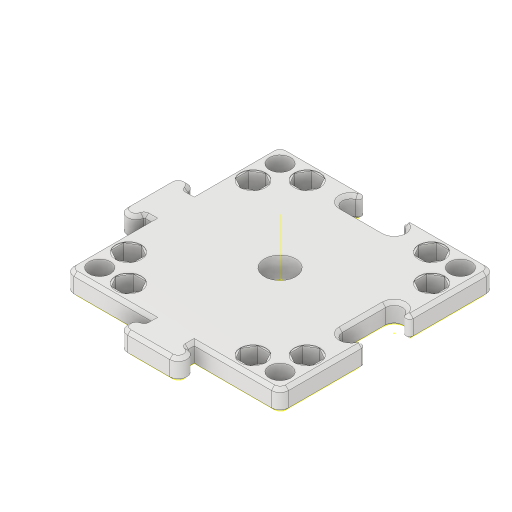
# Autodesk Inventor part: 10_Base_puzzle_syringetip_7.3mm
Saved by Autodesk Inventor 2024.1 (Build 281209000, 209)
## iProperties
Created: 2017-06-20
Part Number: 10_Base_puzzle_syringetip_7.3mm
Material: Generisch
Document SubType Name: Modeling
Designer: diederichbenedict
Density: 1 g/cm^3
Appearance: Weiß
Mass: 5.4697 g
Surface Area: 48.9743 cm^2
Volume: 5.4697 cm^3
Catalog Web Link: isInjectionmolded
Vendor: openUC2
d_part: 50,000 mm
d_o: 40,000 mm
d_i: 40,000 mm
Author: diederichbenedict
Autodesk Inventor part; units mm, degrees
ref_plane "YZ Plane" through (0, 0, 0) normal (1, 0, 0) x (0, 1, 0)
ref_plane "XZ Plane" through (0, 0, 0) normal (0, 1, 0) x (-1, 0, 0)
ref_plane "XY Plane" through (0, 0, 0) normal (0, 0, 1) x (1, 0, 0)
sketch "Skizze1" plane through (0, 0, 0) normal (0, 0, 1) x (1, 0, 0)
  line L0 (-17, 0) -> (-25, 0)
  line L1 (-25, 0) -> (-25, -23)
  line L2 (-23, -25) -> (0, -25)
  line L3 (0, -25) -> (0, -17)
  line L4 (-17, 0) -> (-17, -15)
  line L5 (-15, -17) -> (0, -17)
  arc A0 (-25, -23) -> (-23, -25) centre (-23, -23) ccw
  circle A1 centre (-20.8, -14.5) radius 2.55 construction
  circle A2 centre (-14.5, -20.8) radius 2.55 construction
  arc A3 (-17, -15) -> (-15, -17) centre (-15, -15) ccw
  circle A4 centre (-14.5, -20.8) radius 2.55 construction
  circle A5 centre (-20.8, -14.5) radius 2.55 construction
  line L6 (-30.4971, 0) -> (5.0828, 0) construction
  line L7 (0, -30.4971) -> (0, 5.0828) construction
  line L8 (-18.25, -13.0278) -> (-18.25, -15.9722)
  line L9 (-18.25, -15.9722) -> (-20.8, -17.4445)
  line L10 (-20.8, -17.4445) -> (-23.35, -15.9722)
  line L11 (-23.35, -15.9722) -> (-23.35, -13.0278)
  line L12 (-23.35, -13.0278) -> (-20.8, -11.5555)
  line L13 (-20.8, -11.5555) -> (-18.25, -13.0278)
  line L14 (-15.9722, -18.25) -> (-13.0278, -18.25)
  line L15 (-13.0278, -18.25) -> (-11.5555, -20.8)
  line L16 (-11.5555, -20.8) -> (-13.0278, -23.35)
  line L17 (-13.0278, -23.35) -> (-15.9722, -23.35)
  line L18 (-15.9722, -23.35) -> (-17.4445, -20.8)
  line L19 (-17.4445, -20.8) -> (-15.9722, -18.25)
  point P0 (-25, -25)
  point P1 (-17, -17)
  dimension "d278" = 25
  dimension "d279" = 25
  dimension "d2" = 8
  dimension "d281" = 8
  dimension "d282" = 2
  dimension "d286" = 5.1
  dimension "d_hole" = 5.1
  dimension "d290" = 20.8
  dimension "d" = 20.8
  dimension "d292" = 2
  dimension "d313" = 6.3
  dimension "d314" = 6.3
  dimension "d331" = 0
  dimension "d332" = 0
  constraints: 36 end point, 6 centre point, 6 tangent, 5 coincident, 4 parallel, 4 point on circle, 4 point on line, 2 collinear, 1 horizontal, 1 perpendicular, 26 other
  measures "d278" distance of L2.end point (-25, -25)
  measures "d279" distance of point (-25, -25) L0.end
  measures "d2" distance between parallel lines of L4 L1
  measures "d281" distance between parallel lines of L2 L5
  measures "d282" radius of A0
  measures "d286" diameter of A1
  measures "d_hole" diameter of A2
  measures "d290" distance from line of L0 A2.centre
  measures "d" distance from line of L3 A1.centre
  measures "d292" radius of A3
  measures "d313" horizontal distance of A1.centre A2.centre
  measures "d314" horizontal distance of A1.centre A2.centre
  measures "d331" radial gap between concentric circles of A2 A4
  measures "d332" radial gap between concentric circles of A1 A5
extrude "Extrusion1" add sketch "Skizze1" along normal blind 5
mirror "Mirror6" about plane through (-17, 0, 0) normal (0, 1, 0) of "Extrusion1"
mirror "Mirror7" about plane through (0, -25, 0) normal (1, 0, 0) of "Extrusion1", "Mirror6"
sketch "Sketch26" plane through (0, 0, 5) normal (0, 0, 1) x (1, 0, 0)
  line L0 (23, 25) -> (-23, 25) projected
  arc A0 (-23, 25) -> (-25, 23) centre (-23, 23) ccw projected
  line L1 (-25, -23) -> (-25, 23) projected
  arc A1 (-25, -23) -> (-23, -25) centre (-23, -23) ccw projected
  line L2 (-23, -25) -> (23, -25) projected
  arc A2 (23, -25) -> (25, -23) centre (23, -23) ccw projected
  line L3 (25, 23) -> (25, -23) projected
  arc A3 (25, 23) -> (23, 25) centre (23, 23) ccw projected
  line L4 (15, 17) -> (-15, 17) projected
  arc A4 (17, 15) -> (15, 17) centre (15, 15) ccw projected
  line L5 (17, 15) -> (17, -15) projected
  arc A5 (15, -17) -> (17, -15) centre (15, -15) ccw projected
  line L6 (-15, -17) -> (15, -17) projected
  arc A6 (-17, -15) -> (-15, -17) centre (-15, -15) ccw projected
  line L7 (-17, -15) -> (-17, 15) projected
  arc A7 (-15, 17) -> (-17, 15) centre (-15, 15) ccw projected
  line L8 (-25, -23) -> (-25, 23) projected
  line L9 (-28.6, -6.9) -> (-28.6, -6.9)
  line L10 (-30.6, -4.9) -> (-30.6, 4.9)
  line L11 (-28.6, 6.9) -> (-28.6, 6.9)
  line L12 (-25, 16.8311) -> (-25, -7)
  line L13 (-26.3774, 5) -> (-25, 5)
  line L14 (-25, -5) -> (-26.3774, -5)
  arc A8 (-30.6, -4.9) -> (-28.6, -6.9) centre (-28.6, -4.9) ccw
  arc A9 (-28.6, -6.9) -> (-26.6243, -5.2111) centre (-28.6, -4.9) ccw
  arc A10 (-28.6, 6.9) -> (-30.6, 4.9) centre (-28.6, 4.9) ccw
  arc A11 (-26.6243, 5.2111) -> (-28.6, 6.9) centre (-28.6, 4.9) ccw
  arc A12 (-26.3774, -5) -> (-26.6243, -5.2111) centre (-26.3774, -5.25) ccw
  arc A13 (-26.6243, 5.2111) -> (-26.3774, 5) centre (-26.3774, 5.25) ccw
  line L15 (-42.4199, 0) -> (36.7199, 0) projected
  point P0 (0, 0)
  point P1 (-24.0313, 1.861)
  point P2 (-25, -5)
  point P3 (-25, 5)
  point P4 (-28.6, 6.9)
  dimension "d293" = 5.6
  dimension "d300" = 2
  dimension "d301" = 0.25
  dimension "d365" = 6.9
  dimension "d367" = 6.9
  dimension "d385" = 5
  dimension "d386" = 5
  constraints: 12 end point, 12 point on circle, 10 tangent, 6 centre point, 4 equal radius, 3 parallel, 2 coincident, 2 point on line, 1 horizontal, 1 perpendicular, 1 other
  measures "d293" distance between parallel lines of L1 L10
  measures "d300" radius of A8
  measures "d301" radius of A12
  measures "d385" distance of the line from the sketch origin of L14
  measures "d386" distance of the line from the sketch origin of L13
extrude "Extrusion13" add sketch "Sketch26" against normal up to surface (5 mm away) contours L1 L15 L10 A10 A11 A13 L13 | L1 L14 A12 A9 A8 L10 L15
sketch "Sketch28" plane through (0, 0, 5) normal (0, 0, 1) x (1, 0, 0)
  line L0 (-42.0864, 0) -> (37.3113, 0) construction
  line L1 (23, 25) -> (-23, 25) projected
  arc A0 (-23, 25) -> (-25, 23) centre (-23, 23) ccw projected
  line L2 (-25, 5) -> (-25, 23) projected
  arc A1 (-25, -23) -> (-23, -25) centre (-23, -23) ccw projected
  line L3 (-23, -25) -> (23, -25) projected
  arc A2 (23, -25) -> (25, -23) centre (23, -23) ccw projected
  line L4 (25, 23) -> (25, -23) projected
  arc A3 (25, 23) -> (23, 25) centre (23, 23) ccw projected
  line L5 (15, 17) -> (-15, 17) projected
  arc A4 (17, 15) -> (15, 17) centre (15, 15) ccw projected
  line L6 (17, 15) -> (17, -15) projected
  arc A5 (15, -17) -> (17, -15) centre (15, -15) ccw projected
  line L7 (-15, -17) -> (15, -17) projected
  arc A6 (-17, -15) -> (-15, -17) centre (-15, -15) ccw projected
  line L8 (-17, -15) -> (-17, 15) projected
  arc A7 (-15, 17) -> (-17, 15) centre (-15, 15) ccw projected
  line L9 (24.4624, 5.1058) -> (23.9221, 5.1058) construction
  line L10 (19.1833, 5.0625) -> (23.3833, 5.0625) construction
  line L11 (19.1833, 5.0625) -> (23.3833, 5.0625) construction
  line L12 (23.3833, 5.0625) -> (23.4138, 5.032) construction
  line L13 (23.3833, 5.0625) -> (23.7431, 5.0625) construction
  line L14 (25, 5) -> (25, 0.1058)
  line L15 (25, 23) -> (25, -23) projected
  line L16 (24.4624, 5.1058) -> (25, 5.6434) construction
  line L17 (25, 5) -> (25.2369, 5) construction
  line L18 (25, 5.6434) -> (25, 5)
  line L19 (-25, 5) -> (-26.3774, 5) construction
  arc A8 (-26.6243, 5.2111) -> (-26.3774, 5) centre (-26.3774, 5.25) ccw construction
  arc A9 (-26.6243, 5.2111) -> (-30.6, 4.9) centre (-28.6, 4.9) ccw construction
  line L20 (-30.6, 4.9) -> (-30.6, -4.9) construction
  arc A10 (-30.6, -4.9) -> (-26.6243, -5.2111) centre (-28.6, -4.9) ccw construction
  arc A11 (-26.3774, -5) -> (-26.6243, -5.2111) centre (-26.3774, -5.25) ccw construction
  line L21 (-26.3774, -5) -> (-25, -5) construction
  line L22 (-25, -23) -> (-25, -5) projected
  line L23 (24.4624, -5.1058) -> (23.9221, -5.1058) construction
  line L24 (19.1833, -5.0625) -> (23.3833, -5.0625) construction
  line L25 (19.1833, -5.0625) -> (23.3833, -5.0625) construction
  line L26 (23.3833, -5.0625) -> (23.4138, -5.032) construction
  line L27 (23.3833, -5.0625) -> (23.7431, -5.0625) construction
  line L28 (25, -5) -> (25, 0.1058)
  line L29 (24.4624, -5.1058) -> (25, -5.6434) construction
  line L30 (25, -5) -> (25.2369, -5) construction
  line L31 (25, -5.6434) -> (25, -5)
  line L32 (21.3, -6.95) -> (21.3, -6.95) construction
  line L33 (19.3, -4.95) -> (19.3, 5.05) construction
  line L34 (21.3, 7.05) -> (21.3, 7.05) construction
  line L35 (23.5226, 5.1498) -> (25, 5.1497) construction
  line L36 (25, -5.0501) -> (23.5226, -5.05) construction
  arc A12 (19.3, -4.95) -> (21.3, -6.95) centre (21.3, -4.95) ccw construction
  arc A13 (21.3, -6.95) -> (23.2757, -5.2611) centre (21.3, -4.95) ccw construction
  arc A14 (21.3, 7.05) -> (19.3, 5.05) centre (21.3, 5.05) ccw construction
  arc A15 (23.2757, 5.3609) -> (21.3, 7.05) centre (21.3, 5.05) ccw construction
  arc A16 (23.5226, -5.05) -> (23.2757, -5.2611) centre (23.5226, -5.3) ccw construction
  arc A17 (23.2757, 5.3609) -> (23.5226, 5.1498) centre (23.5226, 5.3998) ccw construction
  line L37 (-30.6, 4.9) -> (-30.6, -4.9) projected
  line L38 (-25, 5) -> (-26.3774, 5) projected
  line L39 (-25, 5) -> (-26.3774, 5)
  arc A18 (-26.6243, 5.2111) -> (-26.3774, 5) centre (-26.3774, 5.25) ccw projected
  arc A19 (-26.6243, 5.2111) -> (-26.3774, 5) centre (-26.3774, 5.25) ccw
  arc A20 (-26.6243, 5.2111) -> (-30.6, 4.9) centre (-28.6, 4.9) ccw
  line L40 (-30.6, 4.9) -> (-30.6, 0)
  line L41 (25, 5.1497) -> (23.4675, 5.1498)
  arc A21 (23.4675, 5.1498) -> (19.55, 5.05) centre (21.51, 5.05) ccw
  line L42 (19.55, 5.05) -> (19.55, 0)
  line L43 (24.4624, -5.1058) -> (23.9221, -5.1058) construction
  line L44 (19.1833, -5.0625) -> (23.3833, -5.0625) construction
  line L45 (19.1833, -5.0625) -> (23.3833, -5.0625) construction
  line L46 (23.3833, -5.0625) -> (23.4138, -5.032) construction
  line L47 (23.3833, -5.0625) -> (23.7431, -5.0625) construction
  line L48 (25, -5) -> (25, -0.1058)
  line L49 (24.4624, -5.1058) -> (25, -5.6434) construction
  line L50 (25, -5) -> (25.2369, -5) construction
  line L51 (25, -5.6434) -> (25, -5)
  arc A22 (23.5226, -5.1498) -> (23.2757, -5.3609) centre (23.5226, -5.3998) ccw construction
  arc A23 (21.3, -7.05) -> (23.2757, -5.3609) centre (21.3, -5.05) ccw construction
  line L52 (23.5226, -5.1498) -> (25, -5.1497) construction
  arc A24 (19.3, -5.05) -> (21.3, -7.05) centre (21.3, -5.05) ccw construction
  line L53 (25, -5.1497) -> (23.4675, -5.1498)
  arc A25 (19.55, -5.05) -> (23.4675, -5.1498) centre (21.51, -5.05) ccw
  arc A26 (23.4675, -5.1498) -> (23.4675, -5.1498) centre (23.3175, -5.15) ccw
  line L54 (19.55, -5.05) -> (19.55, 0)
  line L55 (19.55, 0) -> (25, 0)
  point P0 (23.3495, 5.1058)
  point P1 (23.3495, -5.1058)
  point P2 (25, -7)
  point P3 (25.9687, 1.861)
  point P4 (23.3495, -5.1058)
  point P5 (25.9687, -1.861)
  point P6 (23.4675, -5.1498)
  dimension "d14" = 0
  dimension "d20" = 0
  dimension "d369" = 4.2
  dimension "d370" = 0
  dimension "d380" = 45
  dimension "d387" = 2
  dimension "d388" = 0.25
  dimension "d391" = 0.1
  dimension "d392" = 5.05
  dimension "d393" = 5.05
  dimension "d394" = 1.96
  dimension "d396" = 5.45
  dimension "d397" = 7.05
  constraints: 80 end point, 30 symmetric about line, 28 point on circle, 14 centre point, 14 tangent, 8 point on line, 5 horizontal, 4 collinear, 4 equal radius, 3 coincident, 2 parallel, 2 perpendicular, 1 midpoint, 4 other
  measures "d369" distance of L10.start L10.end
  measures "d370" distance between parallel lines of L10 L11
  measures "d380" angle of L17 L16
  measures "d387" radius of A12
  measures "d388" radius of A16
  measures "d391" distance from line of L35 A15.centre
  measures "d392" distance from line of L0 A15.centre
  measures "d393" distance from line of L0 A21.centre
  measures "d394" radius of A21
  measures "d396" distance between parallel lines of L4 L42
  measures "d397" distance from line of L0 L34.end
extrude "Extrusion14" cut sketch "Sketch28" against normal blind 10 contours L4 L55 L42 A21 L41 | A26 | L4 L53 A25 L54 L55
pattern_circular "Circular Pattern6" count 2 over 90 about axis through (0, 0, 5) along (0, 0, 1) of "Extrusion14", "Extrusion13"
sketch "Sketch29" plane through (0, 0, 5) normal (0, 0, 1) x (1, 0, 0)
  arc A0 (-23, 25) -> (-25, 23) centre (-23, 23) ccw projected
  line L0 (-25, 5) -> (-25, 23) projected
  arc A1 (-25, -23) -> (-23, -25) centre (-23, -23) ccw projected
  line L1 (-23, -25) -> (-5, -25) projected
  arc A2 (23, -25) -> (25, -23) centre (23, -23) ccw projected
  arc A3 (25, 23) -> (23, 25) centre (23, 23) ccw projected
  line L2 (15, 17) -> (-15, 17) projected
  arc A4 (17, 15) -> (15, 17) centre (15, 15) ccw projected
  line L3 (17, 15) -> (17, -15) projected
  arc A5 (15, -17) -> (17, -15) centre (15, -15) ccw projected
  line L4 (-15, -17) -> (15, -17) projected
  arc A6 (-17, -15) -> (-15, -17) centre (-15, -15) ccw projected
  line L5 (-17, -15) -> (-17, 15) projected
  arc A7 (-15, 17) -> (-17, 15) centre (-15, 15) ccw projected
  circle A8 centre (-22, 0) radius 3.89
  circle A9 centre (0, -22) radius 2.9259
  line L6 (-41.9755, 0) -> (36.6458, 0) construction
  line L7 (0, -41.9755) -> (0, 36.6458) construction
  line L8 (25, -5.1497) -> (25, -23) projected
  line L9 (-5.1497, 25) -> (-23, 25) projected
  line L10 (-25, 5) -> (-26.3774, 5) projected
  arc A10 (-26.6243, 5.2111) -> (-26.3774, 5) centre (-26.3774, 5.25) ccw projected
  arc A11 (-26.6243, 5.2111) -> (-30.6, 4.9) centre (-28.6, 4.9) ccw projected
  line L11 (-30.6, 4.9) -> (-30.6, -4.9) projected
  arc A12 (-30.6, -4.9) -> (-26.6243, -5.2111) centre (-28.6, -4.9) ccw projected
  arc A13 (-26.3774, -5) -> (-26.6243, -5.2111) centre (-26.3774, -5.25) ccw projected
  line L12 (-26.3774, -5) -> (-25, -5) projected
  line L13 (-25, -23) -> (-25, -5) projected
  line L14 (-5, -25) -> (-5, -26.3774) projected
  arc A14 (-5.2111, -26.6243) -> (-5, -26.3774) centre (-5.25, -26.3774) ccw projected
  arc A15 (-5.2111, -26.6243) -> (-4.9, -30.6) centre (-4.9, -28.6) ccw projected
  line L15 (-4.9, -30.6) -> (4.9, -30.6) projected
  arc A16 (4.9, -30.6) -> (5.2111, -26.6243) centre (4.9, -28.6) ccw projected
  arc A17 (5, -26.3774) -> (5.2111, -26.6243) centre (5.25, -26.3774) ccw projected
  line L16 (5, -26.3774) -> (5, -25) projected
  line L17 (5, -25) -> (23, -25) projected
  line L18 (-5.1498, 23.4675) -> (-5.1497, 25) projected
  line L19 (25, -5.1497) -> (23.4675, -5.1498) projected
  arc A18 (19.55, -5.05) -> (23.4675, -5.1498) centre (21.51, -5.05) ccw projected
  line L20 (19.55, -5.05) -> (19.55, 5.05) projected
  arc A19 (23.4675, 5.1498) -> (19.55, 5.05) centre (21.51, 5.05) ccw projected
  line L21 (23.4675, 5.1498) -> (25, 5.1497) projected
  line L22 (25, 23) -> (25, 5.1497) projected
  line L23 (23, 25) -> (5.1497, 25) projected
  line L24 (5.1497, 25) -> (5.1498, 23.4675) projected
  arc A20 (5.05, 19.55) -> (5.1498, 23.4675) centre (5.05, 21.51) ccw projected
  line L25 (5.05, 19.55) -> (-5.05, 19.55) projected
  arc A21 (-5.1498, 23.4675) -> (-5.05, 19.55) centre (-5.05, 21.51) ccw projected
  point P0 (0, 0)
  dimension "d319" = 7.78
  dimension "d320" = 5
  dimension "d322" = 5
  constraints: 2 centre point, 2 point on line, 1 coincident
  measures "d319" diameter of A8
  measures "d320" distance from line of A8.centre L5
  measures "d322" distance from line of L4 A9.centre
hole "Hole7" [suppressed]
chamfer "Fase4" [suppressed]
fillet "Rundung5" radius 0.85 8 edges at (25, 5.1497, 2.5) (5.1497, 25, 2.5) (-5.1498, 23.4675, 2.5) (5.1498, 23.4675, 2.5) (23.4675, 5.1498, 2.5) (23.4675, -5.1498, 2.5) (25, -5.1497, 2.5) (-5.1497, 25, 2.5)
sketch "Skizze36" plane through (0, 0, 5) normal (0, 0, 1) x (1, 0, 0)
  line L0 (25, -6.0125) -> (25, -23) projected
  arc A0 (25, 23) -> (23, 25) centre (23, 23) ccw projected
  line L1 (23, 25) -> (6.0125, 25) projected
  line L2 (-6.0125, 25) -> (-5.7214, 25) projected
  line L3 (-6.0125, 25) -> (-23, 25) projected
  arc A1 (-23, 25) -> (-25, 23) centre (-23, 23) ccw projected
  line L4 (-25, 5) -> (-25, 23) projected
  line L5 (-25, 5) -> (-26.3774, 5) projected
  arc A2 (-26.6243, 5.2111) -> (-26.3774, 5) centre (-26.3774, 5.25) ccw projected
  arc A3 (-26.6243, 5.2111) -> (-30.6, 4.9) centre (-28.6, 4.9) ccw projected
  line L6 (-30.6, 4.9) -> (-30.6, -4.9) projected
  arc A4 (-30.6, -4.9) -> (-26.6243, -5.2111) centre (-28.6, -4.9) ccw projected
  arc A5 (-26.3774, -5) -> (-26.6243, -5.2111) centre (-26.3774, -5.25) ccw projected
  line L7 (-26.3774, -5) -> (-25, -5) projected
  line L8 (-25, -23) -> (-25, -5) projected
  arc A6 (-25, -23) -> (-23, -25) centre (-23, -23) ccw projected
  line L9 (-23, -25) -> (-5, -25) projected
  line L10 (-5, -25) -> (-5, -26.3774) projected
  arc A7 (-5.2111, -26.6243) -> (-5, -26.3774) centre (-5.25, -26.3774) ccw projected
  arc A8 (-5.2111, -26.6243) -> (-4.9, -30.6) centre (-4.9, -28.6) ccw projected
  line L11 (-4.9, -30.6) -> (4.9, -30.6) projected
  arc A9 (4.9, -30.6) -> (5.2111, -26.6243) centre (4.9, -28.6) ccw projected
  arc A10 (5, -26.3774) -> (5.2111, -26.6243) centre (5.25, -26.3774) ccw projected
  line L12 (5, -26.3774) -> (5, -25) projected
  line L13 (5, -25) -> (23, -25) projected
  arc A11 (23, -25) -> (25, -23) centre (23, -23) ccw projected
  line L14 (25, 23) -> (25, 6.0125) projected
  line L15 (18.25, 15.9722) -> (20.8, 17.4445) projected
  line L16 (20.8, 17.4445) -> (23.35, 15.9722) projected
  line L17 (23.35, 15.9722) -> (23.35, 13.0278) projected
  line L18 (23.35, 13.0278) -> (20.8, 11.5555) projected
  line L19 (20.8, 11.5555) -> (18.25, 13.0278) projected
  line L20 (18.25, 13.0278) -> (18.25, 15.9722) projected
  line L21 (13.0278, 18.25) -> (11.5555, 20.8) projected
  line L22 (11.5555, 20.8) -> (13.0278, 23.35) projected
  line L23 (13.0278, 23.35) -> (15.9722, 23.35) projected
  line L24 (15.9722, 23.35) -> (17.4445, 20.8) projected
  line L25 (17.4445, 20.8) -> (15.9722, 18.25) projected
  line L26 (15.9722, 18.25) -> (13.0278, 18.25) projected
  line L27 (18.25, -15.9722) -> (20.8, -17.4445) projected
  line L28 (18.25, -13.0278) -> (18.25, -15.9722) projected
  line L29 (20.8, -11.5555) -> (18.25, -13.0278) projected
  line L30 (23.35, -13.0278) -> (20.8, -11.5555) projected
  line L31 (23.35, -15.9722) -> (23.35, -13.0278) projected
  line L32 (20.8, -17.4445) -> (23.35, -15.9722) projected
  line L33 (13.0278, -18.25) -> (11.5555, -20.8) projected
  line L34 (15.9722, -18.25) -> (13.0278, -18.25) projected
  line L35 (17.4445, -20.8) -> (15.9722, -18.25) projected
  line L36 (15.9722, -23.35) -> (17.4445, -20.8) projected
  line L37 (13.0278, -23.35) -> (15.9722, -23.35) projected
  line L38 (11.5555, -20.8) -> (13.0278, -23.35) projected
  line L39 (-18.25, 15.9722) -> (-20.8, 17.4445) projected
  line L40 (-18.25, 13.0278) -> (-18.25, 15.9722) projected
  line L41 (-20.8, 11.5555) -> (-18.25, 13.0278) projected
  line L42 (-23.35, 13.0278) -> (-20.8, 11.5555) projected
  line L43 (-23.35, 15.9722) -> (-23.35, 13.0278) projected
  line L44 (-20.8, 17.4445) -> (-23.35, 15.9722) projected
  line L45 (-13.0278, 18.25) -> (-11.5555, 20.8) projected
  line L46 (-15.9722, 18.25) -> (-13.0278, 18.25) projected
  line L47 (-17.4445, 20.8) -> (-15.9722, 18.25) projected
  line L48 (-15.9722, 23.35) -> (-17.4445, 20.8) projected
  line L49 (-13.0278, 23.35) -> (-15.9722, 23.35) projected
  line L50 (-11.5555, 20.8) -> (-13.0278, 23.35) projected
  line L51 (-13.0278, -18.25) -> (-11.5555, -20.8) projected
  line L52 (-11.5555, -20.8) -> (-13.0278, -23.35) projected
  line L53 (-13.0278, -23.35) -> (-15.9722, -23.35) projected
  line L54 (-15.9722, -23.35) -> (-17.4445, -20.8) projected
  line L55 (-17.4445, -20.8) -> (-15.9722, -18.25) projected
  line L56 (-15.9722, -18.25) -> (-13.0278, -18.25) projected
  line L57 (-18.25, -15.9722) -> (-20.8, -17.4445) projected
  line L58 (-20.8, -17.4445) -> (-23.35, -15.9722) projected
  line L59 (-23.35, -15.9722) -> (-23.35, -13.0278) projected
  line L60 (-23.35, -13.0278) -> (-20.8, -11.5555) projected
  line L61 (-20.8, -11.5555) -> (-18.25, -13.0278) projected
  line L62 (-18.25, -13.0278) -> (-18.25, -15.9722) projected
  line L63 (15, 17) -> (-15, 17) projected
  arc A12 (17, 15) -> (15, 17) centre (15, 15) ccw projected
  line L64 (17, 15) -> (17, -15) projected
  arc A13 (15, -17) -> (17, -15) centre (15, -15) ccw projected
  line L65 (-15, -17) -> (15, -17) projected
  arc A14 (-17, -15) -> (-15, -17) centre (-15, -15) ccw projected
  line L66 (-17, -15) -> (-17, 15) projected
  arc A15 (-15, 17) -> (-17, 15) centre (-15, 15) ccw projected
  circle A16 centre (20.8, 14.5) radius 2.55
  line L67 (18.25, 13.0278) -> (20.8, 11.5555) projected
  circle A17 centre (20.8, -14.5) radius 2.55
  circle A18 centre (20.8, 14.5) radius 2.9445
  line L68 (20.8, -17.4445) -> (18.25, -15.9722) projected
  circle A19 centre (20.8, -14.5) radius 2.9445
  arc A20 (19.55, -5.05) -> (23.3514, -5.7214) centre (21.51, -5.05) ccw projected
  line L69 (19.55, -5.05) -> (19.55, 5.05) projected
  arc A21 (23.3514, 5.7214) -> (19.55, 5.05) centre (21.51, 5.05) ccw projected
  arc A22 (6.0125, 25) -> (5.7214, 23.3514) centre (6.0125, 24.15) ccw projected
  arc A23 (5.05, 19.55) -> (5.7214, 23.3514) centre (5.05, 21.51) ccw projected
  line L70 (5.05, 19.55) -> (-5.05, 19.55) projected
  arc A24 (-5.7214, 23.3514) -> (-5.05, 19.55) centre (-5.05, 21.51) ccw projected
  arc A25 (25, -6.0125) -> (23.3514, -5.7214) centre (24.15, -6.0125) ccw projected
  arc A26 (23.3514, 5.7214) -> (25, 6.0125) centre (24.15, 6.0125) ccw projected
  circle A27 centre (14.5, 20.8) radius 2.55
  circle A28 centre (-14.5, 20.8) radius 2.55
  circle A29 centre (-20.8, 14.5) radius 2.55
  circle A30 centre (-20.8, -14.5) radius 2.55
  circle A31 centre (-14.5, -20.8) radius 2.55
  circle A32 centre (14.5, -20.8) radius 2.55
  point P0 (0, 0)
  constraints: 19 tangent, 8 centre point, 2 coincident, 2 vertical alignment, 4 other
sketch "Skizze37" plane through (0, 0, 5) normal (0, 0, 1) x (1, 0, 0)
  line L0 (25, -6.0125) -> (25, -23) projected
  arc A0 (25, 23) -> (23, 25) centre (23, 23) ccw projected
  line L1 (23, 25) -> (6.0125, 25) projected
  line L2 (-6.0125, 25) -> (-5.7214, 25) projected
  line L3 (-6.0125, 25) -> (-23, 25) projected
  arc A1 (-23, 25) -> (-25, 23) centre (-23, 23) ccw projected
  line L4 (-25, 5) -> (-25, 23) projected
  line L5 (-25, 5) -> (-26.3774, 5) projected
  arc A2 (-26.6243, 5.2111) -> (-26.3774, 5) centre (-26.3774, 5.25) ccw projected
  arc A3 (-26.6243, 5.2111) -> (-30.6, 4.9) centre (-28.6, 4.9) ccw projected
  line L6 (-30.6, 4.9) -> (-30.6, -4.9) projected
  arc A4 (-30.6, -4.9) -> (-26.6243, -5.2111) centre (-28.6, -4.9) ccw projected
  arc A5 (-26.3774, -5) -> (-26.6243, -5.2111) centre (-26.3774, -5.25) ccw projected
  line L7 (-26.3774, -5) -> (-25, -5) projected
  line L8 (-25, -23) -> (-25, -5) projected
  arc A6 (-25, -23) -> (-23, -25) centre (-23, -23) ccw projected
  line L9 (-23, -25) -> (-5, -25) projected
  line L10 (-5, -25) -> (-5, -26.3774) projected
  arc A7 (-5.2111, -26.6243) -> (-5, -26.3774) centre (-5.25, -26.3774) ccw projected
  arc A8 (-5.2111, -26.6243) -> (-4.9, -30.6) centre (-4.9, -28.6) ccw projected
  line L11 (-4.9, -30.6) -> (4.9, -30.6) projected
  arc A9 (4.9, -30.6) -> (5.2111, -26.6243) centre (4.9, -28.6) ccw projected
  arc A10 (5, -26.3774) -> (5.2111, -26.6243) centre (5.25, -26.3774) ccw projected
  line L12 (5, -26.3774) -> (5, -25) projected
  line L13 (5, -25) -> (23, -25) projected
  arc A11 (23, -25) -> (25, -23) centre (23, -23) ccw projected
  line L14 (25, 23) -> (25, 6.0125) projected
  line L15 (13.0278, 18.25) -> (11.5555, 20.8) projected
  line L16 (11.5555, 20.8) -> (13.0278, 23.35) projected
  line L17 (13.0278, 23.35) -> (15.9722, 23.35) projected
  line L18 (15.9722, 23.35) -> (17.4445, 20.8) projected
  line L19 (17.4445, 20.8) -> (15.9722, 18.25) projected
  line L20 (15.9722, 18.25) -> (13.0278, 18.25) projected
  line L21 (13.0278, -18.25) -> (11.5555, -20.8) projected
  line L22 (15.9722, -18.25) -> (13.0278, -18.25) projected
  line L23 (17.4445, -20.8) -> (15.9722, -18.25) projected
  line L24 (15.9722, -23.35) -> (17.4445, -20.8) projected
  line L25 (13.0278, -23.35) -> (15.9722, -23.35) projected
  line L26 (11.5555, -20.8) -> (13.0278, -23.35) projected
  line L27 (-18.25, 15.9722) -> (-20.8, 17.4445) projected
  line L28 (-18.25, 13.0278) -> (-18.25, 15.9722) projected
  line L29 (-20.8, 11.5555) -> (-18.25, 13.0278) projected
  line L30 (-23.35, 13.0278) -> (-20.8, 11.5555) projected
  line L31 (-23.35, 15.9722) -> (-23.35, 13.0278) projected
  line L32 (-20.8, 17.4445) -> (-23.35, 15.9722) projected
  line L33 (-13.0278, 18.25) -> (-11.5555, 20.8) projected
  line L34 (-15.9722, 18.25) -> (-13.0278, 18.25) projected
  line L35 (-17.4445, 20.8) -> (-15.9722, 18.25) projected
  line L36 (-15.9722, 23.35) -> (-17.4445, 20.8) projected
  line L37 (-13.0278, 23.35) -> (-15.9722, 23.35) projected
  line L38 (-11.5555, 20.8) -> (-13.0278, 23.35) projected
  line L39 (-13.0278, -18.25) -> (-11.5555, -20.8) projected
  line L40 (-11.5555, -20.8) -> (-13.0278, -23.35) projected
  line L41 (-13.0278, -23.35) -> (-15.9722, -23.35) projected
  line L42 (-15.9722, -23.35) -> (-17.4445, -20.8) projected
  line L43 (-17.4445, -20.8) -> (-15.9722, -18.25) projected
  line L44 (-15.9722, -18.25) -> (-13.0278, -18.25) projected
  line L45 (-18.25, -15.9722) -> (-20.8, -17.4445) projected
  line L46 (-20.8, -17.4445) -> (-23.35, -15.9722) projected
  line L47 (-23.35, -15.9722) -> (-23.35, -13.0278) projected
  line L48 (-23.35, -13.0278) -> (-20.8, -11.5555) projected
  line L49 (-20.8, -11.5555) -> (-18.25, -13.0278) projected
  line L50 (-18.25, -13.0278) -> (-18.25, -15.9722) projected
  line L51 (15, 17) -> (-15, 17) projected
  arc A12 (17, 15) -> (15, 17) centre (15, 15) ccw projected
  line L52 (17, 15) -> (17, -15) projected
  arc A13 (15, -17) -> (17, -15) centre (15, -15) ccw projected
  line L53 (-15, -17) -> (15, -17) projected
  arc A14 (-17, -15) -> (-15, -17) centre (-15, -15) ccw projected
  line L54 (-17, -15) -> (-17, 15) projected
  arc A15 (-15, 17) -> (-17, 15) centre (-15, 15) ccw projected
  line L55 (-21, 21) -> (21, 21) construction
  line L56 (21, 21) -> (21, -21) construction
  line L57 (21, -21) -> (-21, -21) construction
  line L58 (-21, -21) -> (-21, 21) construction
  line L59 (-21, 21) -> (21, -21) construction
  line L60 (21, 21) -> (-21, -21) construction
  arc A16 (19.55, -5.05) -> (23.3514, -5.7214) centre (21.51, -5.05) ccw projected
  line L61 (19.55, -5.05) -> (19.55, 5.05) projected
  arc A17 (23.3514, 5.7214) -> (19.55, 5.05) centre (21.51, 5.05) ccw projected
  arc A18 (6.0125, 25) -> (5.7214, 23.3514) centre (6.0125, 24.15) ccw projected
  arc A19 (5.05, 19.55) -> (5.7214, 23.3514) centre (5.05, 21.51) ccw projected
  line L62 (5.05, 19.55) -> (-5.05, 19.55) projected
  arc A20 (-5.7214, 23.3514) -> (-5.05, 19.55) centre (-5.05, 21.51) ccw projected
  arc A21 (25, -6.0125) -> (23.3514, -5.7214) centre (24.15, -6.0125) ccw projected
  arc A22 (23.3514, 5.7214) -> (25, 6.0125) centre (24.15, 6.0125) ccw projected
  point P0 (0, 0)
  dimension "d403" = 42
  dimension "d404" = 42
  constraints: 12 end point, 4 coincident, 2 midpoint, 2 parallel, 1 horizontal, 1 perpendicular
  measures "d403" distance of L56.end L57.end
  measures "d404" distance of L55.end L56.end
hole "Bohrung8" at (21, -21, 5) at (-21, -21, 5) at (-21, 21, 5) at (21, 21, 5) direction (0, 0, -1) diameter 5 end through all
chamfer "Fase6" distance 0.75 angle 45 72 edges at (-25, -14, 5) (-24.4142, -24.4142, 5) (-14, -25, 5) (-30.6, 0, 5) (-28.756, -6.8939, 5) (-26.5398, -5.06, 5) (-25.6887, -5, 5) (-28.756, 6.8939, 5) (-26.5398, 5.06, 5) (-25.6887, 5, 5) (-25, 14, 5) (-24.4142, 24.4142, 5) (-14.506, 25, 5) (-5.175, 24.2978, 5) (-6.9802, 21.1693, 5) (0, 19.55, 5) (6.9802, 21.1693, 5) (5.175, 24.2978, 5) (14.506, 25, 5) (24.4142, 24.4142, 5) (25, 14.506, 5) (24.2978, 5.175, 5) (21.1693, 6.9802, 5) (19.55, 0, 5) (21.1693, -6.9802, 5) (24.2978, -5.175, 5) (25, -14.506, 5) (24.4142, -24.4142, 5) (14, -25, 5) (-6.8939, -28.756, 5) (0, -30.6, 5) (6.8939, -28.756, 5) (5.06, -26.5398, 5) (5, -25.6887, 5) (-5.06, -26.5398, 5) (-5, -25.6887, 5) (6.8939, -28.756, 0) (0, -30.6, 0) (-6.8939, -28.756, 0) (-5.06, -26.5398, 0) (-5, -25.6887, 0) (5.06, -26.5398, 0) (5, -25.6887, 0) (14, -25, 0) (24.4142, -24.4142, 0) (25, -14.506, 0) (24.2978, -5.175, 0) (21.1693, -6.9802, 0) (19.55, 0, 0) (21.1693, 6.9802, 0) (24.2978, 5.175, 0) (25, 14.506, 0) (24.4142, 24.4142, 0) (14.506, 25, 0) (5.175, 24.2978, 0) (6.9802, 21.1693, 0) (0, 19.55, 0) (-6.9802, 21.1693, 0) (-5.175, 24.2978, 0) (-14.506, 25, 0) (-24.4142, 24.4142, 0) (-25, 14, 0) (-25, -14, 0) (-24.4142, -24.4142, 0) (-14, -25, 0) (-30.6, 0, 0) (-28.756, 6.8939, 0) (-26.5398, 5.06, 0) (-25.6887, 5, 0) (-28.756, -6.8939, 0) (-26.5398, -5.06, 0) (-25.6887, -5, 0)
hole "Bohrung9" at (20.8, -14.5, 5) at (14.5, -20.8, 5) at (-14.5, -20.8, 5) at (-20.8, -14.5, 5) at (-20.8, 14.5, 5) at (-14.5, 20.8, 5) at (14.5, 20.8, 5) at (20.8, 14.5, 5) direction (0, 0, -1) diameter 6 depth 0.1
sketch "Skizze38" plane through (0, 0, 5) normal (0, 0, 1) x (1, 0, 0)
  circle A0 centre (14.5, 20.8) radius 3 projected
  circle A1 centre (-20.8, 14.5) radius 3 projected
  circle A2 centre (-14.5, -20.8) radius 3 projected
  circle A3 centre (20.8, -14.5) radius 3 projected
  circle A4 centre (14.5, -20.8) radius 3 projected
  circle A5 centre (-20.8, -14.5) radius 3 projected
  circle A6 centre (-14.5, 20.8) radius 3 projected
  circle A7 centre (20.8, 14.5) radius 3 projected
  line L0 (15, 17) -> (-15, 17) projected
  arc A8 (17, 15) -> (15, 17) centre (15, 15) ccw projected
  line L1 (17, 15) -> (17, -15) projected
  arc A9 (15, -17) -> (17, -15) centre (15, -15) ccw projected
  line L2 (-15, -17) -> (15, -17) projected
  arc A10 (-17, -15) -> (-15, -17) centre (-15, -15) ccw projected
  line L3 (-17, -15) -> (-17, 15) projected
  arc A11 (-15, 17) -> (-17, 15) centre (-15, 15) ccw projected
  circle A12 centre (21, 21) radius 2.5 projected
  circle A13 centre (-21, -21) radius 2.5 projected
  circle A14 centre (21, -21) radius 2.5 projected
  circle A15 centre (-21, 21) radius 2.5 projected
  line L4 (-24.25, -23) -> (-24.25, -4.25) projected
  arc A16 (-24.25, -23) -> (-23, -24.25) centre (-23, -23) ccw projected
  line L5 (-4.25, -24.25) -> (-23, -24.25) projected
  line L6 (-4.25, -26.3774) -> (-4.25, -24.25) projected
  arc A17 (-5.0944, -27.3652) -> (-4.25, -26.3774) centre (-5.25, -26.3774) ccw projected
  arc A18 (-5.0944, -27.3652) -> (-4.9, -29.85) centre (-4.9, -28.6) ccw projected
  line L7 (4.9, -29.85) -> (-4.9, -29.85) projected
  arc A19 (4.9, -29.85) -> (5.0944, -27.3652) centre (4.9, -28.6) ccw projected
  arc A20 (4.25, -26.3774) -> (5.0944, -27.3652) centre (5.25, -26.3774) ccw projected
  line L8 (4.25, -24.25) -> (4.25, -26.3774) projected
  line L9 (23, -24.25) -> (4.25, -24.25) projected
  arc A21 (23, -24.25) -> (24.25, -23) centre (23, -23) ccw projected
  line L10 (24.25, -6.0125) -> (24.25, -23) projected
  arc A22 (24.25, -6.0125) -> (24.056, -5.9783) centre (24.15, -6.0125) ccw projected
  arc A23 (18.8, -5.05) -> (24.056, -5.9783) centre (21.51, -5.05) ccw projected
  line L11 (18.8, 5.05) -> (18.8, -5.05) projected
  arc A24 (24.056, 5.9783) -> (18.8, 5.05) centre (21.51, 5.05) ccw projected
  arc A25 (24.056, 5.9783) -> (24.25, 6.0125) centre (24.15, 6.0125) ccw projected
  line L12 (24.25, 23) -> (24.25, 6.0125) projected
  arc A26 (24.25, 23) -> (23, 24.25) centre (23, 23) ccw projected
  line L13 (6.0125, 24.25) -> (23, 24.25) projected
  arc A27 (6.0125, 24.25) -> (5.9783, 24.056) centre (6.0125, 24.15) ccw projected
  arc A28 (5.05, 18.8) -> (5.9783, 24.056) centre (5.05, 21.51) ccw projected
  line L14 (-5.05, 18.8) -> (5.05, 18.8) projected
  arc A29 (-5.9783, 24.056) -> (-5.05, 18.8) centre (-5.05, 21.51) ccw projected
  arc A30 (-5.9783, 24.056) -> (-6.0125, 24.25) centre (-6.0125, 24.15) ccw projected
  line L15 (-23, 24.25) -> (-6.0125, 24.25) projected
  arc A31 (-23, 24.25) -> (-24.25, 23) centre (-23, 23) ccw projected
  line L16 (-24.25, 4.25) -> (-24.25, 23) projected
  line L17 (-26.3774, 4.25) -> (-24.25, 4.25) projected
  arc A32 (-27.3652, 5.0944) -> (-26.3774, 4.25) centre (-26.3774, 5.25) ccw projected
  arc A33 (-27.3652, 5.0944) -> (-29.85, 4.9) centre (-28.6, 4.9) ccw projected
  line L18 (-29.85, -4.9) -> (-29.85, 4.9) projected
  arc A34 (-29.85, -4.9) -> (-27.3652, -5.0944) centre (-28.6, -4.9) ccw projected
  arc A35 (-26.3774, -4.25) -> (-27.3652, -5.0944) centre (-26.3774, -5.25) ccw projected
  line L19 (-24.25, -4.25) -> (-26.3774, -4.25) projected
  point P0 (0, 0)
extrude "Extrusion20" add sketch "Skizze38" against normal blind 5 contours A8 L1 A9 L2 A10 L3 A11 L0
sketch "Skizze39" plane through (0, 0, 5) normal (0, 0, 1) x (1, 0, 0)
  circle A0 centre (14.5, 20.8) radius 3 projected
  circle A1 centre (-20.8, 14.5) radius 3 projected
  circle A2 centre (-14.5, -20.8) radius 3 projected
  circle A3 centre (20.8, -14.5) radius 3 projected
  circle A4 centre (14.5, -20.8) radius 3 projected
  circle A5 centre (-20.8, -14.5) radius 3 projected
  circle A6 centre (-14.5, 20.8) radius 3 projected
  circle A7 centre (20.8, 14.5) radius 3 projected
  circle A8 centre (21, 21) radius 2.5 projected
  circle A9 centre (-21, -21) radius 2.5 projected
  circle A10 centre (21, -21) radius 2.5 projected
  circle A11 centre (-21, 21) radius 2.5 projected
  line L0 (-24.25, -23) -> (-24.25, -4.25) projected
  arc A12 (-24.25, -23) -> (-23, -24.25) centre (-23, -23) ccw projected
  line L1 (-4.25, -24.25) -> (-23, -24.25) projected
  line L2 (-4.25, -26.3774) -> (-4.25, -24.25) projected
  arc A13 (-5.0944, -27.3652) -> (-4.25, -26.3774) centre (-5.25, -26.3774) ccw projected
  arc A14 (-5.0944, -27.3652) -> (-4.9, -29.85) centre (-4.9, -28.6) ccw projected
  line L3 (4.9, -29.85) -> (-4.9, -29.85) projected
  arc A15 (4.9, -29.85) -> (5.0944, -27.3652) centre (4.9, -28.6) ccw projected
  arc A16 (4.25, -26.3774) -> (5.0944, -27.3652) centre (5.25, -26.3774) ccw projected
  line L4 (4.25, -24.25) -> (4.25, -26.3774) projected
  line L5 (23, -24.25) -> (4.25, -24.25) projected
  arc A17 (23, -24.25) -> (24.25, -23) centre (23, -23) ccw projected
  line L6 (24.25, -6.0125) -> (24.25, -23) projected
  arc A18 (24.25, -6.0125) -> (24.056, -5.9783) centre (24.15, -6.0125) ccw projected
  arc A19 (18.8, -5.05) -> (24.056, -5.9783) centre (21.51, -5.05) ccw projected
  line L7 (18.8, 5.05) -> (18.8, -5.05) projected
  arc A20 (24.056, 5.9783) -> (18.8, 5.05) centre (21.51, 5.05) ccw projected
  arc A21 (24.056, 5.9783) -> (24.25, 6.0125) centre (24.15, 6.0125) ccw projected
  line L8 (24.25, 23) -> (24.25, 6.0125) projected
  arc A22 (24.25, 23) -> (23, 24.25) centre (23, 23) ccw projected
  line L9 (6.0125, 24.25) -> (23, 24.25) projected
  arc A23 (6.0125, 24.25) -> (5.9783, 24.056) centre (6.0125, 24.15) ccw projected
  arc A24 (5.05, 18.8) -> (5.9783, 24.056) centre (5.05, 21.51) ccw projected
  line L10 (-5.05, 18.8) -> (5.05, 18.8) projected
  arc A25 (-5.9783, 24.056) -> (-5.05, 18.8) centre (-5.05, 21.51) ccw projected
  arc A26 (-5.9783, 24.056) -> (-6.0125, 24.25) centre (-6.0125, 24.15) ccw projected
  line L11 (-23, 24.25) -> (-6.0125, 24.25) projected
  arc A27 (-23, 24.25) -> (-24.25, 23) centre (-23, 23) ccw projected
  line L12 (-24.25, 4.25) -> (-24.25, 23) projected
  line L13 (-26.3774, 4.25) -> (-24.25, 4.25) projected
  arc A28 (-27.3652, 5.0944) -> (-26.3774, 4.25) centre (-26.3774, 5.25) ccw projected
  arc A29 (-27.3652, 5.0944) -> (-29.85, 4.9) centre (-28.6, 4.9) ccw projected
  line L14 (-29.85, -4.9) -> (-29.85, 4.9) projected
  arc A30 (-29.85, -4.9) -> (-27.3652, -5.0944) centre (-28.6, -4.9) ccw projected
  arc A31 (-26.3774, -4.25) -> (-27.3652, -5.0944) centre (-26.3774, -5.25) ccw projected
  line L15 (-24.25, -4.25) -> (-26.3774, -4.25) projected
  circle A32 centre (0, 0) radius 3.65
  dimension "d427" = 7.3
  constraints: 1 centre point, 1 coincident
  measures "d427" diameter of A32
extrude "Extrusion21" cut sketch "Skizze39" against normal blind 10 contours A32
sketch "Skizze42" plane through (0, 0, 0) normal (0, 0, -1) x (-1, 0, 0)
  circle A0 centre (0, 0) radius 3.65 projected
  line L0 (-20.8, 17.4445) -> (-18.25, 15.9722) projected
  line L1 (-18.25, 15.9722) -> (-18.25, 13.0278) projected
  line L2 (-18.25, 13.0278) -> (-20.8, 11.5555) projected
  line L3 (-20.8, 11.5555) -> (-23.35, 13.0278) projected
  line L4 (-23.35, 13.0278) -> (-23.35, 15.9722) projected
  line L5 (-23.35, 15.9722) -> (-20.8, 17.4445) projected
  line L6 (-11.5555, 20.8) -> (-13.0278, 18.25) projected
  line L7 (-13.0278, 18.25) -> (-15.9722, 18.25) projected
  line L8 (-15.9722, 18.25) -> (-17.4445, 20.8) projected
  line L9 (-17.4445, 20.8) -> (-15.9722, 23.35) projected
  line L10 (-15.9722, 23.35) -> (-13.0278, 23.35) projected
  line L11 (-13.0278, 23.35) -> (-11.5555, 20.8) projected
  line L12 (-20.8, -17.4445) -> (-18.25, -15.9722) projected
  line L13 (-23.35, -15.9722) -> (-20.8, -17.4445) projected
  line L14 (-23.35, -13.0278) -> (-23.35, -15.9722) projected
  line L15 (-20.8, -11.5555) -> (-23.35, -13.0278) projected
  line L16 (-18.25, -13.0278) -> (-20.8, -11.5555) projected
  line L17 (-18.25, -15.9722) -> (-18.25, -13.0278) projected
  line L18 (-11.5555, -20.8) -> (-13.0278, -18.25) projected
  line L19 (-13.0278, -23.35) -> (-11.5555, -20.8) projected
  line L20 (-15.9722, -23.35) -> (-13.0278, -23.35) projected
  line L21 (-17.4445, -20.8) -> (-15.9722, -23.35) projected
  line L22 (-15.9722, -18.25) -> (-17.4445, -20.8) projected
  line L23 (-13.0278, -18.25) -> (-15.9722, -18.25) projected
  line L24 (20.8, 17.4445) -> (18.25, 15.9722) projected
  line L25 (23.35, 15.9722) -> (20.8, 17.4445) projected
  line L26 (23.35, 13.0278) -> (23.35, 15.9722) projected
  line L27 (20.8, 11.5555) -> (23.35, 13.0278) projected
  line L28 (18.25, 13.0278) -> (20.8, 11.5555) projected
  line L29 (18.25, 15.9722) -> (18.25, 13.0278) projected
  line L30 (11.5555, 20.8) -> (13.0278, 18.25) projected
  line L31 (13.0278, 23.35) -> (11.5555, 20.8) projected
  line L32 (15.9722, 23.35) -> (13.0278, 23.35) projected
  line L33 (17.4445, 20.8) -> (15.9722, 23.35) projected
  line L34 (15.9722, 18.25) -> (17.4445, 20.8) projected
  line L35 (13.0278, 18.25) -> (15.9722, 18.25) projected
  line L36 (11.5555, -20.8) -> (13.0278, -18.25) projected
  line L37 (13.0278, -18.25) -> (15.9722, -18.25) projected
  line L38 (15.9722, -18.25) -> (17.4445, -20.8) projected
  line L39 (17.4445, -20.8) -> (15.9722, -23.35) projected
  line L40 (15.9722, -23.35) -> (13.0278, -23.35) projected
  line L41 (13.0278, -23.35) -> (11.5555, -20.8) projected
  line L42 (20.8, -17.4445) -> (18.25, -15.9722) projected
  line L43 (18.25, -15.9722) -> (18.25, -13.0278) projected
  line L44 (18.25, -13.0278) -> (20.8, -11.5555) projected
  line L45 (20.8, -11.5555) -> (23.35, -13.0278) projected
  line L46 (23.35, -13.0278) -> (23.35, -15.9722) projected
  line L47 (23.35, -15.9722) -> (20.8, -17.4445) projected
  circle A1 centre (-21, 21) radius 2.5 projected
  circle A2 centre (21, -21) radius 2.5 projected
  circle A3 centre (-21, -21) radius 2.5 projected
  circle A4 centre (21, 21) radius 2.5 projected
  line L48 (-4.25, -24.25) -> (-23, -24.25) projected
  line L49 (-4.25, -26.3774) -> (-4.25, -24.25) projected
  arc A5 (-5.0944, -27.3652) -> (-4.25, -26.3774) centre (-5.25, -26.3774) ccw projected
  arc A6 (-5.0944, -27.3652) -> (-4.9, -29.85) centre (-4.9, -28.6) ccw projected
  line L50 (4.9, -29.85) -> (-4.9, -29.85) projected
  arc A7 (4.9, -29.85) -> (5.0944, -27.3652) centre (4.9, -28.6) ccw projected
  arc A8 (4.25, -26.3774) -> (5.0944, -27.3652) centre (5.25, -26.3774) ccw projected
  line L51 (4.25, -24.25) -> (4.25, -26.3774) projected
  line L52 (23, -24.25) -> (4.25, -24.25) projected
  arc A9 (23, -24.25) -> (24.25, -23) centre (23, -23) ccw projected
  line L53 (24.25, -4.25) -> (24.25, -23) projected
  line L54 (26.3774, -4.25) -> (24.25, -4.25) projected
  arc A10 (27.3652, -5.0944) -> (26.3774, -4.25) centre (26.3774, -5.25) ccw projected
  arc A11 (27.3652, -5.0944) -> (29.85, -4.9) centre (28.6, -4.9) ccw projected
  line L55 (29.85, 4.9) -> (29.85, -4.9) projected
  arc A12 (29.85, 4.9) -> (27.3652, 5.0944) centre (28.6, 4.9) ccw projected
  arc A13 (26.3774, 4.25) -> (27.3652, 5.0944) centre (26.3774, 5.25) ccw projected
  line L56 (24.25, 4.25) -> (26.3774, 4.25) projected
  line L57 (24.25, 23) -> (24.25, 4.25) projected
  arc A14 (24.25, 23) -> (23, 24.25) centre (23, 23) ccw projected
  line L58 (6.0125, 24.25) -> (23, 24.25) projected
  arc A15 (6.0125, 24.25) -> (5.9783, 24.056) centre (6.0125, 24.15) ccw projected
  arc A16 (5.05, 18.8) -> (5.9783, 24.056) centre (5.05, 21.51) ccw projected
  line L59 (-5.05, 18.8) -> (5.05, 18.8) projected
  arc A17 (-5.9783, 24.056) -> (-5.05, 18.8) centre (-5.05, 21.51) ccw projected
  arc A18 (-5.9783, 24.056) -> (-6.0125, 24.25) centre (-6.0125, 24.15) ccw projected
  line L60 (-23, 24.25) -> (-6.0125, 24.25) projected
  arc A19 (-23, 24.25) -> (-24.25, 23) centre (-23, 23) ccw projected
  line L61 (-24.25, 6.0125) -> (-24.25, 23) projected
  arc A20 (-24.25, 6.0125) -> (-24.056, 5.9783) centre (-24.15, 6.0125) ccw projected
  arc A21 (-18.8, 5.05) -> (-24.056, 5.9783) centre (-21.51, 5.05) ccw projected
  line L62 (-18.8, -5.05) -> (-18.8, 5.05) projected
  arc A22 (-24.056, -5.9783) -> (-18.8, -5.05) centre (-21.51, -5.05) ccw projected
  arc A23 (-24.056, -5.9783) -> (-24.25, -6.0125) centre (-24.15, -6.0125) ccw projected
  line L63 (-24.25, -23) -> (-24.25, -6.0125) projected
  arc A24 (-24.25, -23) -> (-23, -24.25) centre (-23, -23) ccw projected
equation "\"d14\" = 0"
equation "\"d20\" = 0"
equation "\"d_i\" = 40"
equation "\"d_o\" = 40"
equation "\"d_part\" = 50"
equation "\"d6\" = 0"
equation "\"d7\" = 0"
equation "\"d8\" = 0"
equation "\"d9\" = 0"
equation "\"d13\" = 0"
equation "\"d21\" = 0"
equation "\"d22\" = 0"
equation "\"d23\" = 0"
equation "\"d24\" = 0"
equation "\"d25\" = 3"
equation "\"d26\" = 0"
equation "\"d27\" = 0"
equation "\"d28\" = 0"
equation "\"d29\" = 0"
equation "\"d30\" = 0"
equation "\"d31\" = 0"
equation "\"d32\" = 0"
equation "\"d33\" = 0"
equation "\"d34\" = 0"
equation "\"d46\" = 0"
equation "\"d47\" = 0"
equation "\"d48\" = 0"
equation "\"d50\" = 0"
equation "\"d51\" = 0"
equation "\"d52\" = 0"
equation "\"d53\" = 0"
equation "\"d54\" = 0"
equation "\"d55\" = 0"
equation "\"d56\" = 0"
equation "\"d57\" = 0"
equation "\"d58\" = 0"
equation "\"d59\" = 0"
equation "\"magnet_offset\" = 0"
equation "\"screw_offset\" = 0"
equation "\"mal_puzzle_offset\" = 0"
equation "\"fem_puzzle_offset\" = 0"
